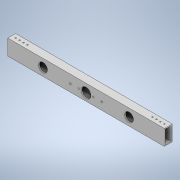
# Autodesk Inventor part: Chassis side 1
Saved by Autodesk Inventor 2022 (Build 260153000, 153)
## iProperties
Created: 2022-11-14
Part Number: Chassis side 1
Material: Generic
Document SubType Name: Modeling
Designer: s135320
Density: 1 g/cm^3
Appearance: Default
Author: s135320
Autodesk Inventor part; units mm, degrees
ref_plane "YZ Plane" through (0, 0, 0) normal (1, 0, 0) x (0, 1, 0)
ref_plane "XZ Plane" through (0, 0, 0) normal (0, 1, 0) x (-1, 0, 0)
ref_plane "XY Plane" through (0, 0, 0) normal (0, 0, 1) x (1, 0, 0)
sketch "Sketch1" plane through (0, 0, 0) normal (0, 1, 0) x (-1, 0, 0)
  point P0 (0, 0)
sketch "Sketch2" plane through (0, 0, 0) normal (0, 0, 1) x (1, 0, 0)
  line L0 (0, 0) -> (508, 0)
  line L1 (508, 0) -> (508, 50.8)
  line L2 (508, 50.8) -> (0, 50.8)
  line L3 (0, 50.8) -> (0, 0)
  circle A0 centre (393.691, 25.4) radius 14.2875
  circle A1 centre (114.309, 25.4) radius 14.2875
  line L4 (0, 25.4) -> (508, 25.4) construction
  line L5 (0, 23.8125) -> (508, 23.8125) construction
  circle A2 centre (254, 23.8125) radius 15.875
  circle A3 centre (230.1875, 23.8125) radius 2.159
  circle A4 centre (277.8125, 23.8125) radius 2.159
  circle A5 centre (304.8, 23.8125) radius 2.54
  circle A6 centre (203.2, 23.8125) radius 2.54
  circle A7 centre (254, 23.8125) radius 139.7 construction
  circle A8 centre (254, 23.8125) radius 23.8125 construction
  dimension "d0" = 50.8
  dimension "d1" = 508
  dimension "d9" = 28.575
  dimension "d10" = 28.575
  dimension "d11" = 1.5875
  dimension "d12" = 279.4
  dimension "d13" = 23.8125
  dimension "d14" = 23.8125
  dimension "d17" = 31.75
  dimension "d18" = 4.318
  dimension "d19" = 4.318
  dimension "d20" = 50.8
  dimension "d21" = 50.8
  dimension "d22" = 5.08
  dimension "d23" = 5.08
  constraints: 12 end point, 8 centre point, 8 point on line, 3 midpoint, 2 coincident, 2 parallel, 2 perpendicular, 2 point on circle, 1 horizontal, 1 horizontal alignment, 2 other
  measures "d0" distance of L2.end L0.start
  measures "d1" distance of L1.end L2.end
  measures "d9" diameter of A0
  measures "d10" diameter of A1
  measures "d11" distance between parallel lines of L4 L5
  measures "d12" diameter of A7
  measures "d13" distance of A4.centre A2.centre
  measures "d14" distance of A2.centre A3.centre
  measures "d17" diameter of A2
  measures "d18" diameter of A3
  measures "d19" diameter of A4
  measures "d20" distance of A2.centre A6.centre
  measures "d21" distance of A5.centre A2.centre
  measures "d22" diameter of A6
  measures "d23" diameter of A5
extrude "Extrusion1" add sketch "Sketch2" along normal blind 25.4 contours L3 L2 L1 L0 | A0 | A1 | A2 | A3 | A4 | A5 | A6
shell "Shell1" thickness 3.175 removed faces 2 at (508, 16.9333, 8.4667) at (0, 33.8667, 16.9333)
extrude "Extrusion2" cut sketch "Sketch2" along normal blind 174.9425 contours A0 | A1 | A2 | A3 | A4 | A5 | A6
sketch "Sketch3" plane through (0, 0, 0) normal (0, 0, -1) x (-1, 0, 0)
  circle A0 centre (-203.2, 23.8125) radius 2.54 projected
  circle A1 centre (-304.8, 23.8125) radius 2.54 projected
  circle A2 centre (-304.8, 23.8125) radius 2.54 projected
  circle A3 centre (-304.8, 23.8125) radius 4.445
  circle A4 centre (-203.2, 23.8125) radius 4.445
  point P0 (0, 0)
  dimension "d29" = 8.89
  dimension "d30" = 8.89
  constraints: 2 centre point, 2 coincident
  measures "d29" diameter of A4
  measures "d30" diameter of A3
extrude "Extrusion3" cut sketch "Sketch3" against normal up to surface (22.225 mm away) contours A0 | A3 | A4
sketch "Sketch4" plane through (0, 50.8, 0) normal (0, 1, 0) x (1, 0, 0)
  line L0 (0, 0) -> (0, -25.4) construction
  line L1 (0, -12.7) -> (508, -12.7) construction
  line L2 (508, -22.225) -> (508, -3.175) construction
  circle A0 centre (12.7, -12.7) radius 2.0701
  circle A1 centre (25.4, -12.7) radius 2.0701
  circle A2 centre (38.1, -12.7) radius 2.0701
  circle A3 centre (50.8, -12.7) radius 2.0701
  line L3 (238.125, -22.225) -> (238.125, -25.4) construction
  line L4 (238.125, -23.8125) -> (238.125, 0) construction
  line L5 (0, -25.4) -> (508, -25.4) construction
  line L6 (254, -25.4) -> (254, 0) construction
  line L7 (238.125, 0) -> (269.875, 0) construction
  circle A4 centre (495.3, -12.7) radius 2.0701
  circle A5 centre (482.6, -12.7) radius 2.0701
  circle A6 centre (469.9, -12.7) radius 2.0701
  circle A7 centre (457.2, -12.7) radius 2.0701
  dimension "d33" = 4.1402
  dimension "d34" = 12.7
  dimension "d37" = 12.7
  constraints: 8 centre point, 6 end point, 5 midpoint, 4 symmetric about line, 1 horizontal, 1 point on line, 1 vertical, 10 other
  measures "d33" diameter of A0
  measures "d34" distance from line of A0.centre L0
  measures "d37" distance of A0.centre A1.centre
extrude "Extrusion4" cut sketch "Sketch4" against normal through all
body "Solid1"
